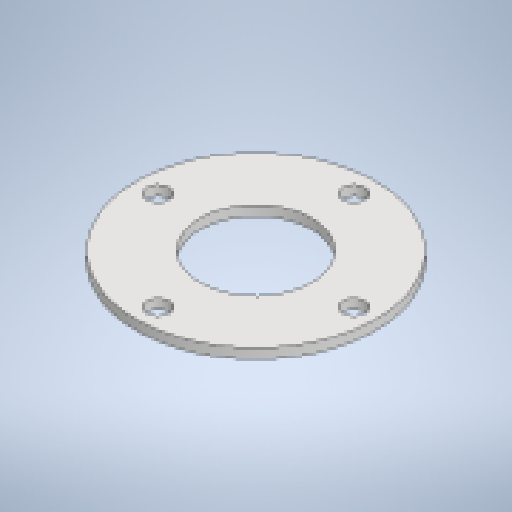
# Autodesk Inventor part: PRS 1200-33 charging blind flange
Saved by Autodesk Inventor 2025.4 (Build 294407000, 407)
## iProperties
Created: 2025-02-13
Part Number: PRS 1200-33 charging blind flange
Material: Steel
Document SubType Name: Sheet Metal
Designer: admin
Mass: 2466.79 g
Surface Area: 934.137 cm^2
Volume: 314.241 cm^3
Density: 7.85 g/cm^3
Flat Pattern Width: 19.5 cm
Flat Pattern Length: 19.5 cm
Flat Pattern Area: 380.25 cm^2
Sheet Metal Rule: AISI304 4mm Die 32
Sheet Metal Width: 195,000 mm
Sheet Metal Length: 195,000 mm
Sheet Metal Area: 38025,000 mm^2
Appearance: Default
Author: pokla
Autodesk Inventor part; units mm, degrees
ref_plane "YZ Plane" through (0, 0, 0) normal (1, 0, 0) x (0, 1, 0)
ref_plane "XZ Plane" through (0, 0, 0) normal (0, 1, 0) x (-1, 0, 0)
ref_plane "XY Plane" through (0, 0, 0) normal (0, 0, 1) x (1, 0, 0)
sketch "Sketch2" plane through (0, 0, 0) normal (0, 0, 1) x (1, 0, 0)
  circle A0 centre (0, 0) radius 45.5
  circle A1 centre (0, 0) radius 97.5
  circle A2 centre (0, 0) radius 80 construction
  circle A3 centre (80, 0) radius 9
  circle A4 centre (0, 80) radius 9
  circle A5 centre (-80, 0) radius 9
  circle A6 centre (0, -80) radius 9
  dimension "D_b_c" = 160
  dimension "D_min" = 91
  dimension "D_max" = 195
  dimension "Blt_hl" = 18
  dimension "d33" = 360
  measures "D_min" diameter of A0
  measures "D_max" diameter of A1
  measures "Blt_hl" diameter of A3
extrude "Plate2" add sketch "Sketch2" along normal blind 8
equation "\"d14\" = Thickness"
equation "\"BendReliefWidth\" = Thickness"
equation "\"BendReliefDepth\" = 0.5 * Thickness"
equation "\"CornerReliefSize\" = 4 * Thickness"
equation "\"MinimumRemnant\" = 2 * Thickness"
equation "\"TransitionRadius\" = BendRadius"
equation "\"JacobiRadiusSize\" = BendRadius"
equation "\"GapSize\" = Thickness"
equation "\"Thickness\" = 8"
equation "\"BendRadius\" = 6"
body "Solid3"
